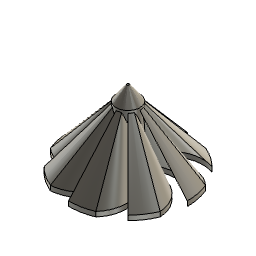
jet_turbine (Autodesk Fusion 360 design; units mm, degrees)
Autodesk Fusion 360 part; units mm, degrees
sketch "Sketch3" plane through (0, 0, 0) normal (0, 0, 1) x (1, 0, 0)
  circle A0 centre (0, 0) radius 125
  dimension "d12" = 250
  constraint coincident A0.centre origin
  measures "d12" diameter of A0
extrude "Extrude2" add sketch "Sketch3" along normal blind 10 makes body 1
sketch "Sketch4" plane through (0, 0, 10) normal (0, 0, 1) x (-1, 0, 0)
  circle A0 centre (0, 0) radius 125
  line L0 (0, 0) -> (0, -125) construction
  arc A1 (0, 0) -> (0, -125) centre (80, -62.5) ccw
  arc A2 (0, 0) -> (88.3883, -88.3883) centre (100.7627, 12.3744) ccw
  arc A3 (0, 0) -> (125, 0) centre (62.5, 80) ccw
  arc A4 (0, 0) -> (88.3883, 88.3883) centre (-12.3744, 100.7627) ccw
  arc A5 (0, 0) -> (0, 125) centre (-80, 62.5) ccw
  arc A6 (0, 0) -> (-88.3883, 88.3883) centre (-100.7627, -12.3744) ccw
  arc A7 (0, 0) -> (-125, 0) centre (-62.5, -80) ccw
  arc A8 (0, 0) -> (-88.3883, -88.3883) centre (12.3744, -100.7627) ccw
  dimension "d15" = 80
  dimension "d17" = 360
  constraint coincident A0.centre L0.start
  constraint coincident A0 L0.end
  constraint vertical L0
  measures "d15" distance of L0 A1.centre
sketch "Sketch5" plane through (0, 0, 0) normal (0, 0, 1) x (1, 0, 0)
  circle A0 centre (0, 0) radius 25
  dimension "d18" = 50
  constraint coincident A0.centre origin
  measures "d18" diameter of A0
extrude "Extrude3" add sketch "Sketch5" along normal blind 5 separate body makes body 2
move_body "Move2" bodies 2 to x (1, 0, 0) y (0, 1, 0) z (0, 0, 1) at (0, 0, 100)
move_body "Move3" bodies 2 to x (1, 0, 0) y (0, 1, 0) z (0, 0, 1) at (0, 0, 25)
sketch "Sketch6" plane through (0, 0, 0) normal (0, 0, 1) x (1, 0, 0)
  circle A0 centre (0, 0) radius 2.5
  dimension "d21" = 5
  constraint coincident A0.centre origin
  measures "d21" diameter of A0
extrude "Extrude4" add sketch "Sketch6" along normal blind 1 separate body makes body 3
move_body "Move4" bodies 3 to x (1, 0, 0) y (0, 1, 0) z (0, 0, 1) at (0, 0, 175)
move_body "Move5" bodies 3 to x (1, 0, 0) y (0, 1, 0) z (0, 0, 1) at (0, 0, -15)
loft "Loft1" add section 1 face at (-0.8863, 0.2321, 160) section 2 face at (-6.7759, -1.242, 130) on bodies 2 3 bodies 2 3
fillet "Fillet1" radius 2.5 1 edges at (-2.3308, -0.904, 161) on bodies 2 3
sketch "Sketch7" plane through (0, 0, 10) normal (0, 0, 1) x (-1, 0, 0)
  circle A0 centre (0, 0) radius 125
  line L0 (0, 0) -> (0, 125) construction
  arc A1 (0, 125) -> (0, 0) centre (30, 62.5) ccw
  arc A2 (-47.8354, 115.4849) -> (0, 0) centre (3.7987, 69.223) ccw
  arc A3 (-88.3883, 88.3883) -> (0, 0) centre (-22.981, 65.4074) ccw
  arc A4 (-115.4849, 47.8354) -> (0, 0) centre (-46.262, 51.6341) ccw
  arc A5 (-125, 0) -> (0, 0) centre (-62.5, 30) ccw
  arc A6 (-115.4849, -47.8354) -> (0, 0) centre (-69.223, 3.7987) ccw
  arc A7 (-88.3883, -88.3883) -> (0, 0) centre (-65.4074, -22.981) ccw
  arc A8 (-47.8354, -115.4849) -> (0, 0) centre (-51.6341, -46.262) ccw
  arc A9 (0, -125) -> (0, 0) centre (-30, -62.5) ccw
  arc A10 (47.8354, -115.4849) -> (0, 0) centre (-3.7987, -69.223) ccw
  arc A11 (88.3883, -88.3883) -> (0, 0) centre (22.981, -65.4074) ccw
  arc A12 (115.4849, -47.8354) -> (0, 0) centre (46.262, -51.6341) ccw
  arc A13 (125, 0) -> (0, 0) centre (62.5, -30) ccw
  arc A14 (115.4849, 47.8354) -> (0, 0) centre (69.223, -3.7987) ccw
  arc A15 (88.3883, 88.3883) -> (0, 0) centre (65.4074, 22.981) ccw
  arc A16 (47.8354, 115.4849) -> (0, 0) centre (51.6341, 46.262) ccw
  dimension "d35" = 30
  dimension "d37" = 360
  constraint coincident A0.centre L0.start
  constraint coincident A0 L0.end
  constraint vertical L0
  measures "d35" distance of L0 A1.centre
sketch "Sketch8" plane through (0, 0, 125) normal (0, 0, -1) x (1, 0, 0)
  circle A0 centre (0, 0) radius 25
  line L0 (0, -25) -> (0, 0) construction
  line L1 (0, 0) -> (9.5671, -23.097) construction
  line L2 (4.7835, -11.5485) -> (-15.219, -19.8338) construction
  arc A1 (0, 0) -> (9.5671, -23.097) centre (23.2611, -3.8948) ccw
  arc A2 (0, 0) -> (17.6777, -17.6777) centre (22.981, 5.3033) ccw
  arc A3 (0, 0) -> (23.097, -9.5671) centre (19.2022, 13.694) ccw
  arc A4 (0, 0) -> (25, 0) centre (12.5, 20) ccw
  arc A5 (0, 0) -> (23.097, 9.5671) centre (3.8948, 23.2611) ccw
  arc A6 (0, 0) -> (17.6777, 17.6777) centre (-5.3033, 22.981) ccw
  arc A7 (0, 0) -> (9.5671, 23.097) centre (-13.694, 19.2022) ccw
  arc A8 (0, 0) -> (0, 25) centre (-20, 12.5) ccw
  arc A9 (0, 0) -> (-9.5671, 23.097) centre (-23.2611, 3.8948) ccw
  arc A10 (0, 0) -> (-17.6777, 17.6777) centre (-22.981, -5.3033) ccw
  arc A11 (0, 0) -> (-23.097, 9.5671) centre (-19.2022, -13.694) ccw
  arc A12 (0, 0) -> (-25, 0) centre (-12.5, -20) ccw
  arc A13 (0, 0) -> (-23.097, -9.5671) centre (-3.8948, -23.2611) ccw
  arc A14 (0, 0) -> (-17.6777, -17.6777) centre (5.3033, -22.981) ccw
  arc A15 (0, 0) -> (-9.5671, -23.097) centre (13.694, -19.2022) ccw
  arc A16 (0, 0) -> (0, -25) centre (20, -12.5) ccw
  dimension "d30" = 22.5
  dimension "d31" = 20
  dimension "d33" = 360
  constraint coincident A0 L0.start
  constraint coincident A0.centre L0.end
  constraint vertical L0
  constraint coincident A0 L1.end
  constraint midpoint L1 L2.start
  constraint coincident A0 L2.end
  constraint perpendicular L1 L2
  measures "d30" angle of L0 L1
  measures "d31" distance of L1 A1.centre
loft "Loft2" add profiles "Sketch7", "Sketch8" section 1 contours A0 A13 A14 section 2 contours A0 A11 A12 bodies 1
loft "Loft3" add profiles "Sketch8", "Sketch7" section 1 contours A0 A13 A14 section 2 contours A0 A11 A12 separate body makes body 4
loft "Loft4" add profiles "Sketch8", "Sketch7" section 1 contours A0 A15 A16 section 2 contours A0 A9 A10 separate body makes body 5
loft "Loft5" add profiles "Sketch8", "Sketch7" section 1 contours A0 A1 A2 section 2 contours A0 A7 A8 separate body makes body 6
loft "Loft6" add profiles "Sketch8", "Sketch7" section 1 contours A0 A3 A4 section 2 contours A0 A5 A6 separate body makes body 7
loft "Loft7" add profiles "Sketch8", "Sketch7" section 1 contours A0 A5 A6 section 2 contours A0 A3 A4 separate body makes body 8
loft "Loft8" add profiles "Sketch7", "Sketch8" section 1 contours A0 A1 A2 section 2 contours A0 A7 A8 separate body makes body 9
loft "Loft9" add profiles "Sketch7", "Sketch8" section 1 contours A0 A15 A16 section 2 contours A0 A9 A10 separate body makes body 10
extrude "Extrude5" cut sketch "Sketch7" against normal blind 10 contours A0 A12 A13 | A0 A14 A15 | A0 A2 A3 | A0 A4 A5 | A0 A6 A7 | A0 A8 A9 | A0 A10 A11 | A0 A1 A16 bodies 1
extrude "Extrude6" add 1 faces at (-6.7759, -1.242, 125) along direction (0, 0, -1) blind 125 on bodies 2 bodies 1 2 4 5 6 7 8 9 10
